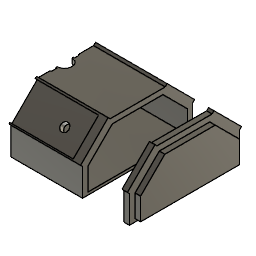
gorlov+case (Autodesk Fusion 360 design; units mm, degrees)
Autodesk Fusion 360 part; units mm, degrees
note: some values were not read from the file. Set by a fixed rule: which sketch regions a step uses.
sketch "Sketch1" plane through (0, 0, 0) normal (0, 0, 1) x (1, 0, 0)
  line L0 (-130, 0) -> (170, 0)
  line L1 (170, 0) -> (170, 200)
  line L2 (170, 200) -> (-130, 200)
  line L3 (-130, 200) -> (-130, 0)
  dimension "d1" = 300
  dimension "d2" = 200
  constraint horizontal L0
  constraint vertical L1
  constraint horizontal L2
  constraint vertical L3
  measures "d1" distance of L0.start L0.end
  measures "d2" distance of L0.start L2.end
extrude "Extrude1" add sketch "Sketch1" along normal blind 225 makes body 1
chamfer "Chamfer1" distance 50 angle 45 1 edges at (20, 0, 225) on bodies 1
chamfer "Chamfer2" distance 50 angle 45 1 edges at (20, 200, 225) on bodies 1
extrude "Extrude2" cut 1 faces at (-30, 133.3333, 0) along direction (0, 0, 1) blind 50 on bodies 1 bodies 1
move_body "Move1" bodies 1 to x (1, 0, 0) y (0, 1, 0) z (0, 0, 1) at (0, 0, -50)
move_body "Move2" bodies 1 to x (1, 0, 0) y (0, 1, 0) z (0, 0, 1) at (-20, -100, 0)
shell "Shell1" thickness 10 removed faces 1 at (150, -33.3333, 41.6667) on bodies 1
sketch "Sketch2" plane through (150, 0, 0) normal (1, 0, 0) x (0, 1, 0)
  line L0 (90, 10) -> (-90, 10)
  line L1 (-90, 10) -> (-90, 120.8579)
  line L2 (-90, 120.8579) -> (-45.8579, 165)
  line L3 (-45.8579, 165) -> (45.8579, 165)
  line L4 (45.8579, 165) -> (90, 120.8579)
  line L5 (90, 120.8579) -> (90, 10)
  line L6 (-100, 0) -> (100, 0)
  line L7 (100, 0) -> (100, 125)
  line L8 (100, 125) -> (50, 175)
  line L9 (50, 175) -> (-50, 175)
  line L10 (-50, 175) -> (-100, 125)
  line L11 (-100, 125) -> (-100, 0)
  line L12 (-45.8579, 165) -> (45.8579, 165)
  line L13 (90, 120.8579) -> (90, 10)
  line L14 (-90, 10) -> (-90, 120.8579)
  line L15 (-45.8579, 165) -> (-90, 120.8579)
  line L16 (-90, 10) -> (90, 10)
  line L17 (45.8579, 165) -> (90, 120.8579)
  constraint coincident L2.end L3.start
  constraint coincident L3.end L4.start
  constraint coincident L4.end L5.start
  constraint coincident L0.start L5.end
  constraint coincident L0.end L1.start
  constraint coincident L1.end L2.start
extrude "Extrude3" cut sketch "Sketch2" against normal blind 430 contours L0 L1 L2 L3 L4 L5 L12 L13 L14 L15 L16 L17 bodies 1
sketch "Sketch3" plane through (0, 0, 10) normal (0, 0, 1) x (-1, 0, 0)
  line L0 (150, 90) -> (-150, 90)
  line L1 (-150, 90) -> (-150, -90)
  line L2 (-150, -90) -> (150, -90)
  line L3 (150, -90) -> (150, 90)
sketch "Sketch4" plane through (0, 0, 175) normal (0, 0, 1) x (-1, 0, 0)
  line L0 (-150, -50) -> (150, -50)
  line L1 (150, -50) -> (150, 50)
  line L2 (150, 50) -> (-150, 50)
  line L3 (-150, 50) -> (-150, -50)
  circle A0 centre (0, 2.5) radius 13.4181
  circle A1 centre (0, -16) radius 2.1265
  circle A2 centre (0, 20.5) radius 2.1793
extrude "Extrude4" cut sketch "Sketch4" against normal blind 11 contours A0 | A1 | A2 bodies 1
sketch "Sketch5" plane through (0, 112.5, 112.5) normal (0, 0.707107, 0.707107) x (-1, 0, 0)
  line L0 (150, 17.6777) -> (150, 88.3883)
  line L1 (150, 88.3883) -> (-150, 88.3883)
  line L2 (-150, 88.3883) -> (-150, 17.6777)
  line L3 (-150, 17.6777) -> (150, 17.6777)
  line L4 (-135, 85) -> (-20, 85)
  line L5 (-20, 85) -> (-20, 20)
  line L6 (-20, 20) -> (-135, 20)
  line L7 (-135, 20) -> (-135, 85)
  line L8 (135, 85) -> (20, 85)
  line L9 (20, 85) -> (20, 20)
  line L10 (20, 20) -> (135, 20)
  line L11 (135, 20) -> (135, 85)
  constraint horizontal L4
  constraint vertical L5
  constraint horizontal L6
  constraint vertical L7
  constraint horizontal L8
  constraint vertical L9
  constraint horizontal L10
  constraint vertical L11
extrude "Extrude5" add sketch "Sketch5" along normal blind 5 bodies 1
sketch "Sketch6" plane through (0, -112.5, 112.5) normal (0, -0.707107, 0.707107) x (1, 0, 0)
  line L0 (150, 17.6777) -> (150, 88.3883)
  line L1 (150, 88.3883) -> (-150, 88.3883)
  line L2 (-150, 88.3883) -> (-150, 17.6777)
  line L3 (-150, 17.6777) -> (150, 17.6777)
  line L4 (-135, 85) -> (-20, 85)
  line L5 (-20, 85) -> (-20, 20)
  line L6 (-20, 20) -> (-135, 20)
  line L7 (-135, 20) -> (-135, 85)
  line L8 (135, 85) -> (20, 85)
  line L9 (20, 85) -> (20, 20)
  line L10 (20, 20) -> (135, 20)
  line L11 (135, 20) -> (135, 85)
  constraint horizontal L4
  constraint vertical L5
  constraint horizontal L6
  constraint vertical L7
  constraint horizontal L8
  constraint vertical L9
  constraint horizontal L10
  constraint vertical L11
extrude "Extrude6" add sketch "Sketch6" along normal blind 5 bodies 1
sketch "Sketch7" plane through (0, 0, 0) normal (1, 0, 0) x (0, 1, 0)
sketch "Sketch8" plane through (-150, 0, 0) normal (-1, 0, 0) x (0, -1, 0)
  line L0 (90, 120.8579) -> (90, 10)
  line L1 (90, 10) -> (-90, 10)
  line L2 (-90, 10) -> (-90, 120.8579)
  line L3 (-90, 120.8579) -> (-45.8579, 165)
  line L4 (-45.8579, 165) -> (45.8579, 165)
  line L5 (45.8579, 165) -> (90, 120.8579)
  line L6 (-100, 0) -> (100, 0)
  line L7 (100, 0) -> (100, 125)
  line L8 (100, 125) -> (103.5355, 128.5355)
  line L9 (103.5355, 128.5355) -> (53.5355, 178.5355)
  line L10 (53.5355, 178.5355) -> (50, 175)
  line L11 (50, 175) -> (-50, 175)
  line L12 (-50, 175) -> (-53.5355, 178.5355)
  line L13 (-53.5355, 178.5355) -> (-103.5355, 128.5355)
  line L14 (-103.5355, 128.5355) -> (-100, 125)
  line L15 (-100, 125) -> (-100, 0)
  line L16 (-45.8579, 165) -> (45.8579, 165)
  line L17 (90, 120.8579) -> (90, 10)
  line L18 (90, 120.8579) -> (45.8579, 165)
  line L19 (-45.8579, 165) -> (-90, 120.8579)
  line L20 (-90, 120.8579) -> (-90, 10)
  line L21 (90, 10) -> (-90, 10)
  line L22 (53.5355, 178.5355) -> (103.5355, 128.5355)
  line L23 (100, 125) -> (103.5355, 128.5355)
  line L24 (100, 125) -> (100, 0)
  line L25 (100, 0) -> (-100, 0)
  line L26 (-100, 125) -> (-100, 0)
  line L27 (-100, 125) -> (-103.5355, 128.5355)
  line L28 (-103.5355, 128.5355) -> (-53.5355, 178.5355)
  line L29 (-53.5355, 178.5355) -> (-50, 175)
  line L30 (-50, 175) -> (50, 175)
  line L31 (50, 175) -> (53.5355, 178.5355)
  constraint coincident L3.end L4.start
  constraint coincident L4.end L5.start
  constraint coincident L0.start L5.end
  constraint coincident L0.end L1.start
  constraint coincident L2.end L3.start
  constraint coincident L1.end L2.start
  constraint coincident L9.end L10.start
  constraint coincident L8.end L9.start
  constraint coincident L7.end L8.start
  constraint coincident L6.end L7.start
  constraint coincident L6.start L15.end
  constraint coincident L14.end L15.start
  constraint coincident L13.end L14.start
  constraint coincident L12.end L13.start
  constraint coincident L11.end L12.start
  constraint coincident L10.end L11.start
extrude "Extrude7" add sketch "Sketch8" along normal blind 15 separate body contours L0 L1 L2 L3 L4 L5 L16 L17 L18 L19 L20 L21 makes body 2
extrude "Extrude8" add 1 faces at (-150, -82.357, 142.643) along direction (-1, 0, 0) blind 10 separate body on bodies 1 makes body 3
move_body "Move3" bodies 3 2 to x (1, 0, 0) y (0, 1, 0) z (0, 0, 1) at (-60, 0, 0)
extrude "Extrude9" add 1 faces at (-225, 30, 83.9052) along direction (-1, 0, 0) blind 5 on bodies 2 bodies 2
sketch "Sketch9" plane through (0, 0, 175) normal (0, 0, 1) x (-1, 0, 0)
  circle A0 centre (0, 2.5) radius 13.4181
  circle A1 centre (0, 20.5) radius 2.1793
  circle A2 centre (0, -16) radius 2.1265
  line L0 (-150, -50) -> (150, -50)
  line L1 (150, -50) -> (150, 50)
  line L2 (150, 50) -> (-150, 50)
  line L3 (-150, 50) -> (-150, -50)
move_body "Move4" bodies 3 2 to x (-1, 0, 0) y (0, -1, 0) z (0, 0, 1) at (-440, -3.5355, 0)
extrude "Extrude10" cut 1 faces at (-223.3333, -78.8215, 135.5719) along direction (0, 0.707107, -0.707107) blind 0.5 on bodies 2 bodies 2
extrude "Extrude11" cut 1 faces at (-223.3333, -93.5355, 46.9526) along direction (0, 1, 0) blind 0.5 on bodies 2 bodies 2
extrude "Extrude12" cut 1 faces at (-216.6667, 57.0364, 150.286) along direction (0, -0.707107, -0.707107) blind 0.5 on bodies 2 bodies 2
extrude "Extrude13" cut 1 faces at (-223.3333, 86.4645, 83.9052) along direction (0, -1, 0) blind 0.5 on bodies 2 bodies 2
extrude "Extrude14" cut 1 faces at (-223.3333, 26.2978, 10) along direction (0, 0, 1) blind 0.5 on bodies 2 bodies 2
extrude "Extrude15" cut 1 faces at (-223.3333, -93.0355, 47.2169) along direction (0, 1, 0) blind 0.5 on bodies 2 bodies 2
extrude "Extrude16" cut 1 faces at (-223.3333, -18.8215, 165) along direction (0, 0, -1) blind 0.5 on bodies 2 bodies 2
extrude "Extrude17" add 1 faces at (-223.3333, -92.5355, 47.2169) along direction (0, -1, 0) blind 0.5 on bodies 2 bodies 2
extrude "Extrude18" add 1 faces at (-226.6667, -33.5355, 10) along direction (0, 0, 1) blind 130 on bodies 3 bodies 2 3
extrude "Extrude19" add 1 faces at (-226.6667, -57.7267, 156.6667) along direction (0, 0.707107, -0.707107) blind 52 on bodies 2 bodies 2
extrude "Extrude20" add 1 faces at (-226.6667, 58.989, 148.3333) along direction (0, -0.707107, -0.707107) blind 18 on bodies 2 bodies 2
extrude "Extrude21" add 1 faces at (-226.6667, 11.7504, 165) along direction (0, 0, -1) blind 31 on bodies 2 bodies 2
extrude "Extrude22" cut 1 faces at (-150, -82.357, 142.643) along direction (1, 0, 0) blind 150 on bodies 1 bodies 1
extrude "Extrude23" cut 1 faces at (-230, 29.7978, 83.3333) along direction (1, 0, 0) blind 40 on bodies 2 bodies 2
sketch "Sketch10" plane through (0, 112.5, 112.5) normal (0, 0.707107, 0.707107) x (-1, 0, 0)
  line L0 (-20, 20) -> (-20, 85)
  line L1 (-20, 85) -> (-135, 85)
  line L2 (-135, 85) -> (-135, 20)
  line L3 (-135, 20) -> (-20, 20)
  circle A0 centre (-75, 50) radius 7.5
  dimension "d52" = 15
  measures "d52" diameter of A0
extrude "Extrude24" cut sketch "Sketch10" against normal blind 10 contours A0 bodies 1
sketch "Sketch11" plane through (0, -112.5, 112.5) normal (0, -0.707107, 0.707107) x (1, 0, 0)
  line L0 (135, 85) -> (20, 85)
  line L1 (20, 85) -> (20, 20)
  line L2 (20, 20) -> (135, 20)
  line L3 (135, 20) -> (135, 85)
  circle A0 centre (75, 50) radius 7.5
  dimension "d55" = 15
  measures "d55" diameter of A0
extrude "Extrude25" cut sketch "Sketch11" against normal blind 15 contours A0 bodies 1
extrude "Extrude26" cut 1 faces at (150, -67.643, 157.357) along direction (-1, 0, 0) blind 10 on bodies 1 bodies 1
extrude "Extrude27" cut 1 faces at (20, 70.0736, 159.6405) along direction (-1, 0, 0) blind 10 on bodies 1 bodies 1
extrude "Extrude28" add 1 faces at (135, 68.8951, 158.4619) along direction (-1, 0, 0) blind 10 on bodies 1 bodies 1 2
extrude "Extrude29" cut 1 faces at (140, -67.643, 157.357) along direction (-1, 0, 0) blind 10 on bodies 1 bodies 1
sketch "Sketch12" plane through (0, -112.5, 112.5) normal (0, -0.707107, 0.707107) x (1, 0, 0)
  line L0 (130, 20) -> (130, 85)
  line L1 (130, 85) -> (20, 85)
  line L2 (20, 85) -> (20, 20)
  line L3 (20, 20) -> (130, 20)
  circle A0 centre (75, 50) radius 7.5
  line L4 (130, 85) -> (125, 85)
  line L5 (125, 85) -> (125, 20)
  line L6 (125, 20) -> (130, 20)
  line L7 (130, 20) -> (130, 85)
  constraint horizontal L4
  constraint vertical L5
  constraint horizontal L6
  constraint vertical L7
  constraint coincident L3 L5.end
  constraint coincident L0.end L1.start
extrude "Extrude30" add sketch "Sketch12" along normal blind 5 contours L0 L1 L3 L4 L5 L6 L7 bodies 1
extrude "Extrude31" cut 1 faces at (10, 70.0736, 159.6405) along direction (-1, 0, 0) blind 5 on bodies 1 bodies 1
extrude "Extrude32" add 1 faces at (125, 68.8951, 158.4619) along direction (-1, 0, 0) blind 5 on bodies 1 bodies 1
extrude "Extrude33" add 1 faces at (125, -84.2157, 143.1413) along direction (-1, 0, 0) blind 5 on bodies 1 bodies 1
extrude "Extrude34" cut 1 faces at (20, -70.0736, 159.6405) along direction (-1, 0, 0) blind 5 on bodies 1 bodies 1
extrude "Extrude35" add 1 faces at (120, -84.2157, 143.1413) along direction (-1, 0, 0) blind 5 on bodies 1 bodies 1
extrude "Extrude36" cut 1 faces at (15, -70.0736, 159.6405) along direction (-1, 0, 0) blind 10 on bodies 1 bodies 1
extrude "Extrude37" cut 1 faces at (115, -84.2157, 143.1413) along direction (1, 0, 0) blind 5 on bodies 1 bodies 1
extrude "Extrude38" cut 1 faces at (5, -70.0736, 159.6405) along direction (-1, 0, 0) blind 5 on bodies 1 bodies 1
extrude "Extrude39" add 1 faces at (120, -84.2157, 143.1413) along direction (-1, 0, 0) blind 5 on bodies 1 bodies 1
extrude "Extrude40" add 1 faces at (120, 68.8951, 158.4619) along direction (-1, 0, 0) blind 5 on bodies 1 bodies 1
extrude "Extrude41" cut 1 faces at (5, 70.0736, 159.6405) along direction (-1, 0, 0) blind 10 on bodies 1 bodies 1
extrude "Extrude42" cut 1 faces at (86.6667, -33.3333, 0) along direction (0, 0, 1) blind 25 on bodies 1 bodies 1
sketch "Sketch13" plane through (0, -90, 0) normal (0, 1, 0) x (-1, 0, 0)
  line L0 (-130, 25) -> (0, 25)
  line L1 (0, 25) -> (0, 120.8579)
  line L2 (0, 120.8579) -> (-130, 120.8579)
  line L3 (-130, 120.8579) -> (-130, 25)
  line L4 (-130, 25) -> (0, 25)
  line L5 (0, 25) -> (0, 30)
  line L6 (0, 30) -> (-130, 30)
  line L7 (-130, 30) -> (-130, 25)
  constraint horizontal L4
  constraint vertical L5
  constraint horizontal L6
  constraint vertical L7
  constraint coincident L1 L5.end
  constraint coincident L0.start L3.end
extrude "Extrude43" add sketch "Sketch13" along normal blind 180 contours L0 L1 L3 L4 L5 L6 L7 bodies 1
extrude "Extrude44" cut 1 faces at (43.3333, 33.3333, 25) along direction (0, 0, 1) blind 25 on bodies 1 bodies 1
sketch "Sketch14" plane through (0, -90, 0) normal (0, 1, 0) x (-1, 0, 0)
  line L0 (-130, 50) -> (0, 50)
  line L1 (0, 50) -> (0, 120.8579)
  line L2 (0, 120.8579) -> (-130, 120.8579)
  line L3 (-130, 120.8579) -> (-130, 50)
  line L4 (-130, 50) -> (2.4482, 50)
  line L5 (2.4482, 50) -> (2.4482, 55)
  line L6 (2.4482, 55) -> (-130, 55)
  line L7 (-130, 55) -> (-130, 50)
  dimension "d96" = 5
  constraint horizontal L4
  constraint vertical L5
  constraint horizontal L6
  constraint vertical L7
  constraint coincident L0.start L3.end
  measures "d96" distance of L0.start L6.end
extrude "Extrude45" add sketch "Sketch14" along normal blind 180 contours L0 L1 L3 L4 L6 L7 bodies 1
extrude "Extrude46" cut 1 faces at (43.3333, 33.3333, 50) along direction (0, 0, 1) blind 25 on bodies 1 bodies 1
sketch "Sketch15" plane through (0, -90, 0) normal (0, 1, 0) x (-1, 0, 0)
  line L0 (-130, 75) -> (0, 75)
  line L1 (0, 75) -> (0, 120.8579)
  line L2 (0, 120.8579) -> (-130, 120.8579)
  line L3 (-130, 120.8579) -> (-130, 75)
  line L4 (0, 75) -> (-130, 75)
  line L5 (-130, 75) -> (-130, 80)
  line L6 (-130, 80) -> (0, 80)
  line L7 (0, 80) -> (0, 75)
  constraint horizontal L4
  constraint vertical L5
  constraint horizontal L6
  constraint vertical L7
  constraint coincident L3 L5.end
  constraint coincident L0.end L1.start
extrude "Extrude47" add sketch "Sketch15" along normal blind 180 contours L0 L1 L3 L4 L5 L6 L7 bodies 1
sketch "Sketch16" plane through (130, 0, 0) normal (1, 0, 0) x (0, 1, 0)
  line L0 (-100, 75) -> (100, 75)
  line L1 (100, 75) -> (100, 125)
  line L2 (100, 125) -> (103.5355, 128.5355)
  line L3 (103.5355, 128.5355) -> (53.5355, 178.5355)
  line L4 (53.5355, 178.5355) -> (50, 175)
  line L5 (50, 175) -> (-50, 175)
  line L6 (-50, 175) -> (-53.5355, 178.5355)
  line L7 (-53.5355, 178.5355) -> (-103.5355, 128.5355)
  line L8 (-103.5355, 128.5355) -> (-100, 125)
  line L9 (-100, 125) -> (-100, 75)
  line L10 (90, 80) -> (-90, 80)
  line L11 (-90, 80) -> (-90, 120.8579)
  line L12 (-90, 120.8579) -> (-45.8579, 165)
  line L13 (-45.8579, 165) -> (45.8579, 165)
  line L14 (45.8579, 165) -> (90, 120.8579)
  line L15 (90, 120.8579) -> (90, 80)
extrude "Extrude48" add sketch "Sketch16" along normal blind 10 separate body makes body 4
sketch "Sketch17" plane through (140, 0, 0) normal (1, 0, 0) x (0, 1, 0)
  line L0 (45.8579, 165) -> (90, 120.8579)
  line L1 (90, 120.8579) -> (90, 80)
  line L2 (90, 80) -> (-90, 80)
  line L3 (-90, 80) -> (-90, 120.8579)
  line L4 (-90, 120.8579) -> (-45.8579, 165)
  line L5 (-45.8579, 165) -> (45.8579, 165)
  line L6 (-100, 125) -> (-100, 75)
  line L7 (-100, 75) -> (100, 75)
  line L8 (100, 75) -> (100, 125)
  line L9 (100, 125) -> (103.5355, 128.5355)
  line L10 (103.5355, 128.5355) -> (53.5355, 178.5355)
  line L11 (53.5355, 178.5355) -> (50, 175)
  line L12 (50, 175) -> (-50, 175)
  line L13 (-50, 175) -> (-53.5355, 178.5355)
  line L14 (-53.5355, 178.5355) -> (-103.5355, 128.5355)
  line L15 (-103.5355, 128.5355) -> (-100, 125)
extrude "Extrude49" add sketch "Sketch17" along normal blind 10 separate body contours L0 L1 L2 L3 L4 L5 makes body 5
move_body "Move5" bodies 4 5 to x (1, 0, 0) y (0, 1, 0) z (0, 0, 1) at (75, 0, 0)
extrude "Extrude50" add 1 faces at (215, 15.286, 108.3333) along direction (-1, 0, 0) blind 10 on bodies 5 bodies 4 5
extrude "Extrude51" cut 1 faces at (221.6667, 75.286, 135.5719) along direction (0, -0.707107, -0.707107) blind 0.25 on bodies 4 bodies 4
extrude "Extrude52" cut 1 faces at (218.3333, -15.286, 165) along direction (0, 0, -1) blind 0.25 on bodies 4 bodies 4
extrude "Extrude53" cut 1 faces at (218.3333, -75.286, 135.5719) along direction (0, 0.707107, -0.707107) blind 0.25 on bodies 4 bodies 4
extrude "Extrude54" cut 1 faces at (218.3333, -90, 93.6193) along direction (0, 1, 0) blind 0.25 on bodies 4 bodies 4
extrude "Extrude55" cut 1 faces at (221.6667, 90, 93.6193) along direction (0, -1, 0) blind 0.25 on bodies 4 bodies 4
extrude "Extrude56" cut 1 faces at (221.6667, 29.9167, 80) along direction (0, 0, 1) blind 0.25 on bodies 4 bodies 4
extrude "Extrude57" cut 1 faces at (218.3333, -15.2514, 164.75) along direction (0, 0, -1) blind 0.1 on bodies 4 bodies 4
extrude "Extrude58" cut 1 faces at (221.6667, -60.4195, 150.0848) along direction (0, 0.707107, -0.707107) blind 0.1 on bodies 4 bodies 4
extrude "Extrude59" cut 1 faces at (221.6667, 60.4195, 150.0848) along direction (0, -0.707107, -0.707107) blind 0.1 on bodies 4 bodies 4
extrude "Extrude60" cut 1 faces at (221.6667, 89.75, 107.2529) along direction (0, -1, 0) blind 0.1 on bodies 4 bodies 4
extrude "Extrude61" cut 1 faces at (218.3333, -89.75, 93.7514) along direction (0, 1, 0) blind 0.1 on bodies 4 bodies 4
extrude "Extrude62" cut 1 faces at (218.3333, 29.8833, 80.25) along direction (0, 0, 1) blind 0.1 on bodies 4 bodies 4
sketch "Sketch18" plane through (0, 0, 0) normal (-1, 0, 0) x (0, -1, 0)
  line L0 (-100, 75) -> (100, 75)
  line L1 (100, 75) -> (100, 125)
  line L2 (100, 125) -> (103.5355, 128.5355)
  line L3 (103.5355, 128.5355) -> (101.8934, 130.1777)
  line L4 (101.8934, 130.1777) -> (98.3579, 126.6421)
  line L5 (98.3579, 126.6421) -> (52.3959, 172.6041)
  line L6 (52.3959, 172.6041) -> (55.9315, 176.1396)
  line L7 (55.9315, 176.1396) -> (53.5355, 178.5355)
  line L8 (53.5355, 178.5355) -> (50, 175)
  line L9 (50, 175) -> (22.6793, 175)
  line L10 (22.6793, 175) -> (22.6793, 165)
  line L11 (22.6793, 165) -> (45.8579, 165)
  line L12 (45.8579, 165) -> (90, 120.8579)
  line L13 (90, 120.8579) -> (90, 80)
  line L14 (90, 80) -> (-90, 80)
  line L15 (-90, 80) -> (-90, 120.8579)
  line L16 (-90, 120.8579) -> (-45.8579, 165)
  line L17 (-45.8579, 165) -> (-18.1265, 165)
  line L18 (-18.1265, 165) -> (-18.1265, 175)
  line L19 (-18.1265, 175) -> (-50, 175)
  line L20 (-50, 175) -> (-53.5355, 178.5355)
  line L21 (-53.5355, 178.5355) -> (-55.9315, 176.1396)
  line L22 (-55.9315, 176.1396) -> (-52.3959, 172.6041)
  line L23 (-52.3959, 172.6041) -> (-98.3579, 126.6421)
  line L24 (-98.3579, 126.6421) -> (-101.8934, 130.1777)
  line L25 (-101.8934, 130.1777) -> (-103.5355, 128.5355)
  line L26 (-103.5355, 128.5355) -> (-100, 125)
  line L27 (-100, 125) -> (-100, 75)
  circle A0 centre (95, 115) radius 2.5
  circle A1 centre (95, 90) radius 2.5
  circle A2 centre (-95, 115) radius 2.5
  circle A3 centre (-95, 90) radius 2.5
  circle A4 centre (-35, 170) radius 2.5
  circle A5 centre (34.2686, 169.2117) radius 2.5
  dimension "d133" = 5
  dimension "d134" = 5
  dimension "d135" = 5
  dimension "d136" = 5
  dimension "d137" = 5
  dimension "d138" = 5
  measures "d133" diameter of A0
  measures "d134" diameter of A1
  measures "d135" diameter of A2
  measures "d136" diameter of A3
  measures "d137" diameter of A4
  measures "d138" diameter of A5
extrude "Extrude63" cut sketch "Sketch18" against normal blind 10 contours A0 | A1 | A2 | A3 | A4 | A5 bodies 1
sketch "Sketch19" plane through (0, 0, 175) normal (0, 0, 1) x (-1, 0, 0)
  line L0 (-130, 50) -> (-130, -50)
  line L1 (-130, -50) -> (0, -50)
  line L2 (0, -50) -> (0, -18.1265)
  arc A0 (0, -13.8735) -> (0, -18.1265) centre (0, -16) ccw
  line L3 (0, -13.8735) -> (0, -10.9181)
  arc A1 (0, 15.9181) -> (0, -10.9181) centre (0, 2.5) ccw
  line L4 (0, 15.9181) -> (0, 18.3208)
  arc A2 (0, 22.6793) -> (0, 18.3208) centre (0, 20.5) ccw
  line L5 (0, 22.6793) -> (0, 50)
  line L6 (0, 50) -> (-130, 50)
  line L7 (-2.1265, -16) -> (-2.1265, -27.3064)
  line L8 (-2.1265, -27.3064) -> (-2.1265, 31)
  circle A3 centre (0, -21) radius 2.1265
  circle A4 centre (0, -18.8735) radius 2.1265
  circle A5 centre (0, 27) radius 2.1265
  circle A6 centre (0, 24) radius 2.1265
  line L9 (0, 18.3208) -> (-2.1265, 18.3208)
  line L10 (-2.1265, 18.3208) -> (-2.1265, 27)
  line L11 (-2.1265, 27) -> (0, 27)
  line L12 (0, 27) -> (0, 18.3208)
  line L13 (0, -13.8735) -> (-2.1265, -13.8735)
  line L14 (-2.1265, -13.8735) -> (-2.1265, -21)
  line L15 (-2.1265, -21) -> (0, -21)
  line L16 (0, -21) -> (0, -13.8735)
  constraint midpoint A0 L7.start
  constraint tangent A0 L7
  constraint parallel L2 L7
  constraint parallel L2 L8
  constraint coincident L2 A3.centre
  constraint tangent L7 A3
  constraint coincident L2 A4.centre
  constraint coincident A3 A4.centre
  constraint tangent L7 A4
  constraint coincident L5 A5.centre
  constraint tangent L8 A5
  constraint coincident L5 A6.centre
  constraint tangent L8 A6
  constraint horizontal L9
  constraint vertical L10
  constraint horizontal L11
  constraint vertical L12
  constraint coincident A5 L10.end
  constraint coincident L8 L10.end
  constraint coincident L4.end A2.end
  constraint horizontal L13
  constraint vertical L14
  constraint horizontal L15
  constraint vertical L16
  constraint coincident L8 L14.end
  constraint coincident A3 L14.end
  constraint coincident A0.start L3.start
extrude "Extrude64" cut sketch "Sketch19" against normal blind 10 contours L5 A5 L11 | L2 A3 L15 | L5 A5 A6 L11 L12 | L8 A5 A6 L10 | L2 A3 A4 L16 | A3 A4 L15 | L7 L8 A3 A4 L14 | L5 A5 A6 L12 | A2 L8 A6 L10 | A2 L5 A5 A6 L12 | L2 A0 A3 A4 L16 | A0 L7 L8 A4 L14 | A2 L8 A6 L10 L12 | A2 A6 L12 | A0 A4 L16 | A0 L8 L13 L14 | A0 A4 L16 | A2 L8 L9 L10 picked at (-0.1056, -20.2832) picked at (-0.0928, 25.7027) bodies 1
